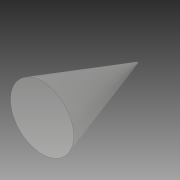
# Autodesk Inventor part: Sichtkegel 25 Grad
Saved by Autodesk Inventor 2019.4 (Build 234330000, 330)
## iProperties
Part Number: Sichtkegel 25 Grad
Material: Generisch
Document SubType Name: Modeling
Designer: rYan
Density: 1 g/cm^3
Appearance: Klar - hell
Author: rYan
Autodesk Inventor part; units mm, degrees
ref_plane "YZ Plane" through (0, 0, 0) normal (1, 0, 0) x (0, 1, 0)
ref_plane "XZ Plane" through (0, 0, 0) normal (0, 1, 0) x (-1, 0, 0)
ref_plane "XY Plane" through (0, 0, 0) normal (0, 0, 1) x (1, 0, 0)
sketch "Skizze1" plane through (0, 0, 0) normal (1, 0, 0) x (0, 1, 0)
  line L0 (0, 0) -> (-50, 0)
  line L1 (-50, 0) -> (-50, 16.496)
  line L2 (-50, 16.496) -> (0, 0.25)
  line L3 (0, 0.25) -> (0, 0)
  dimension "d0" = 18
  dimension "d1" = 50
  dimension "d3" = 0.5
  constraints: 8 end point, 1 horizontal, 1 perpendicular, 1 vertical
  measures "d0" angle of L0 L2
  measures "d1" distance from line of L0.start L1
  measures "d3" diameter of L2.end L0
revolve "Umdrehung1" add sketch "Skizze1" angle 360 about axis through (0, 0, 0) along (0, -1, 0)
